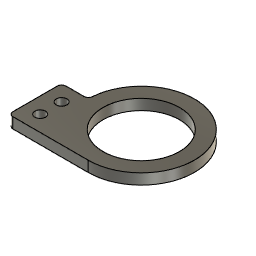
Random-part (Autodesk Fusion 360 design; units mm, degrees)
Autodesk Fusion 360 part; units mm, degrees
sketch "Sketch1" plane through (0, 0, 0) normal (0, 0, 1) x (1, 0, 0)
  line L0 (0, 0) -> (-75, 0)
  line L1 (-75, 0) -> (-75, 50)
  line L2 (-75, 50) -> (-50, 50)
  arc A0 (0, 0) -> (-50, 50) centre (0, 50) ccw
  constraint horizontal L0
  constraint vertical L1
  constraint horizontal L2
  constraint coincident L0.start A0.start
extrude "Extrude1" add sketch "Sketch1" along normal blind 10
fillet "Fillet1" radius 4 3 edges at (-75, 0, 5) (-75, 50, 5) (-50, 50, 5)
hole "Hole1" at (0, 50, 10) direction (0, 0, -1) diameter 72 depth 10 tip angle 118
hole "Hole2" at (-60.0592, 35.0034, 10) direction (0, 0, -1) diameter 10 depth 10 tip angle 118
hole "Hole3" at (-60.1262, 14.9013, 10) direction (0, 0, -1) diameter 10 depth 10 tip angle 118
